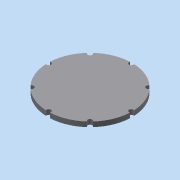
# Autodesk Inventor part: tapa
Saved by Autodesk Inventor 2015 (Build 190159000, 159)
## iProperties
Created: 2017-10-02
Part Number: tapa
Material: Generic
Document SubType Name: Modeling
Designer: macbook
Density: 1 g/cm^3
Appearance: Default
Author: macbook
Autodesk Inventor part; units mm, degrees
ref_plane "YZ Plane" through (0, 0, 0) normal (1, 0, 0) x (0, 1, 0)
ref_plane "XZ Plane" through (0, 0, 0) normal (0, 1, 0) x (-1, 0, 0)
ref_plane "XY Plane" through (0, 0, 0) normal (0, 0, 1) x (1, 0, 0)
sketch "Sketch1" plane through (0, 0, 0) normal (0, 0, 1) x (1, 0, 0)
  circle A0 centre (0, 0) radius 47.5
  circle A1 centre (46.5, 0) radius 2.5
  dimension "d0" = 95
  dimension "d1" = 5
  constraints: 2 centre point, 1 coincident
  measures "d0" diameter of A0
  measures "d1" diameter of A1
extrude "Extrusion1" add sketch "Sketch1" along normal blind 5.5 contours A0 A1 | A1 A0 picked at (46.4291, -0.6491) picked at (-16.8425, 0)
sketch "Sketch2" plane through (0, 0, 5.5) normal (0, 0, 1) x (1, 0, 0)
  circle A0 centre (46.5, 0) radius 2.5
  circle A1 centre (32.8805, 32.8805) radius 2.5
  circle A2 centre (0, 46.5) radius 2.5
  circle A3 centre (-32.8805, 32.8805) radius 2.5
  circle A4 centre (-46.5, 0) radius 2.5
  circle A5 centre (-32.8805, -32.8805) radius 2.5
  circle A6 centre (0, -46.5) radius 2.5
  circle A7 centre (32.8805, -32.8805) radius 2.5
  point P0 (0, 0)
  dimension "d4" = 5
  dimension "d7" = 360
  constraints: 8 centre point, 17 other
  measures "d4" diameter of A0
extrude "Extrusion2" cut sketch "Sketch2" against normal blind 5.5
body "Solid1"
